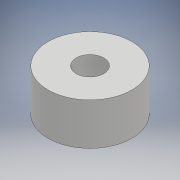
# Autodesk Inventor part: 磁鐵
Saved by Autodesk Inventor 2018 (Build 220112000, 112)
## iProperties
Created: 2025-10-22
Part Number: 磁鐵
Material: 一般
Document SubType Name: Modeling
Designer: User
Density: 1 g/cm^3
Appearance: 預設
Author: User
Autodesk Inventor part; units mm, degrees
ref_plane "YZ Plane" through (0, 0, 0) normal (1, 0, 0) x (0, 1, 0)
ref_plane "XZ Plane" through (0, 0, 0) normal (0, 1, 0) x (-1, 0, 0)
ref_plane "XY Plane" through (0, 0, 0) normal (0, 0, 1) x (1, 0, 0)
sketch "草圖1" plane through (0, 0, 0) normal (0, 0, 1) x (1, 0, 0)
  circle A0 centre (0, 0) radius 7.3
  circle A1 centre (0, 0) radius 22.2
  dimension "d0" = 44.4
  dimension "d1" = 14.6
  constraints: 2 centre point, 2 coincident
  measures "d0" diameter of A1
  measures "d1" diameter of A0
extrude "擠出1" add sketch "草圖1" along normal blind 22.25
